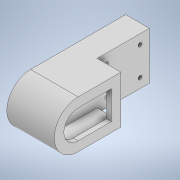
# Autodesk Inventor part: Link2_v2a
Saved by Autodesk Inventor 2022 (Build 260153000, 153)
## iProperties
Created: 2022-06-07
Part Number: Link2_v2a
Material: Generic
Document SubType Name: Modeling
Designer: Asus
Density: 1 g/cm^3
Appearance: Default
Author: Asus
Autodesk Inventor part; units mm, degrees
ref_plane "YZ Plane" through (0, 0, 0) normal (1, 0, 0) x (0, 1, 0)
ref_plane "XZ Plane" through (0, 0, 0) normal (0, 1, 0) x (-1, 0, 0)
ref_plane "XY Plane" through (0, 0, 0) normal (0, 0, 1) x (1, 0, 0)
sketch "Sketch1" plane through (0, 0, 0) normal (1, 0, 0) x (0, 1, 0)
  line L0 (25, 22.5) -> (-25, 22.5)
  line L1 (-25, 22.5) -> (-25, -100)
  line L2 (-25, -100) -> (25, -100)
  line L3 (25, -100) -> (25, 22.5)
  circle A0 centre (0, 0) radius 25
  circle A1 centre (0, 0) radius 20
  circle A2 centre (0, 0) radius 3.2936
  point P0 (25, 0)
  point P1 (-25, 0)
  dimension "d0" = 50
  dimension "d1" = 122.5
  dimension "d2" = 25
  dimension "d3" = 22.5
  dimension "d12" = 40
  dimension "d13" = 6.5872
  constraints: 8 end point, 3 centre point, 3 coincident, 2 parallel, 1 horizontal, 1 perpendicular, 1 tangent
  measures "d0" distance of L1.end L2.end
  measures "d1" distance of L0.end L1.end
  measures "d2" distance from line of L3 point (0, 0)
  measures "d3" distance from line of L0 point (0, 0)
  measures "d12" diameter of A1
  measures "d13" diameter of A2
extrude "Extrusion1" add sketch "Sketch1" along normal blind 5 contours A0 L0 | L0 A0 | L3 L2 L1 A0 | A1
sketch "Sketch4" plane through (5, 0, 0) normal (1, 0, 0) x (0, 0, -1)
  line L0 (100, -25) -> (100, 25) projected
  line L1 (100, 25) -> (0, 25) projected
  line L2 (100, -25) -> (0, -25)
  line L3 (0, -25) -> (0, 25)
  line L4 (0, 25) -> (100, 25)
  line L5 (100, 25) -> (100, -25)
  circle A0 centre (0, 0) radius 3.2936 projected
  arc A1 (15, 20) -> (15, -20) centre (0, 0) ccw
  circle A2 centre (0, 0) radius 20
  line L6 (0, 20) -> (95, 20)
  line L7 (95, 20) -> (95, -20)
  line L8 (95, -20) -> (0, -20)
  line L9 (0, -20) -> (0, 20)
  point P0 (0, -20)
  dimension "d15" = 40
  dimension "d14" = 50
  dimension "d16" = 5
  dimension "d17" = 5
  constraints: 16 end point, 4 parallel, 3 point on line, 2 coincident, 2 horizontal, 2 perpendicular, 2 point on circle, 1 centre point, 3 other
  measures "d14" diameter of A1
  measures "d16" distance between parallel lines of L2 L8
  measures "d17" distance between parallel lines of L0 L7
extrude "Extrusion3" add sketch "Sketch4" along normal blind 45 contours L2 A1 L8 L7 L6 L1 L0 | A1 L3 A2 | L3 L8 A1 | A1 L6 L3
sketch "Sketch5" plane through (50, 0, 0) normal (1, 0, 0) x (0, 0, -1)
  line L0 (100, -25) -> (100, 25) projected
  line L1 (0, 25) -> (100, 25)
  line L2 (100, 25) -> (100, -25)
  line L3 (100, -25) -> (0, -25)
  line L4 (0, -25) -> (0, 25)
  circle A0 centre (0, 0) radius 25
  arc A1 (0, 20) -> (0, -20) centre (0, 0) ccw projected
  circle A2 centre (0, 0) radius 15
  line L5 (0, 15) -> (35, 15)
  line L6 (35, 15) -> (35, -15)
  line L7 (35, -15) -> (0, -15)
  line L8 (0, -15) -> (0, 15)
  point P0 (0, -15)
  point P1 (100, 25)
  dimension "d20" = 30
  dimension "d21" = 10
  dimension "d22" = 50
  dimension "d23" = 35
  constraints: 16 end point, 4 parallel, 2 coincident, 2 horizontal, 2 perpendicular, 1 centre point, 1 point on line, 3 other
  measures "d21" distance between parallel lines of L3 L7
  measures "d22" diameter of A0
  measures "d23" distance from line of point (0, 0) L6
extrude "Extrusion4" add sketch "Sketch5" against normal blind 5 contours L3 A0 L7 L6 L5 L1 L0 | A0 L4 A1 | L4 L7 A0 | A0 L5 L4 | A1 L4 A2
sketch "Sketch6" plane through (5, 0, 0) normal (1, 0, 0) x (0, 0, -1)
  circle A0 centre (0, 0) radius 20
  line L0 (95, 20) -> (0, 20) projected
  line L1 (0, -20) -> (95, -20) projected
  line L2 (0, 20) -> (22, 20)
  line L3 (22, 20) -> (22, -20)
  line L4 (22, -20) -> (0, -20)
  line L5 (0, -20) -> (0, 20)
  dimension "d26" = 22
  constraints: 8 end point, 2 parallel, 1 centre point, 1 coincident, 1 horizontal, 1 perpendicular, 1 point on line
  measures "d26" distance between parallel lines of L3 L5
extrude "Extrusion5" add sketch "Sketch6" along normal blind 20
sketch "Sketch7" plane through (0, 0, 0) normal (-1, 0, 0) x (0, 0, 1)
  circle A0 centre (0, 0) radius 9.5
  dimension "d29" = 19
  constraints: 1 centre point, 1 coincident
  measures "d29" diameter of A0
extrude "Extrusion6" cut sketch "Sketch7" against normal blind 12.5
sketch "Sketch8" plane through (0, 0, 0) normal (-1, 0, 0) x (0, 0, 1)
  circle A0 centre (0, 0) radius 11.5
  dimension "d32" = 23
  constraints: 1 centre point, 1 coincident
  measures "d32" diameter of A0
extrude "Extrusion7" cut sketch "Sketch8" against normal blind 6.5
sketch "Sketch9" plane through (12.5, 0, 0) normal (-1, 0, 0) x (0, 0, 1)
  circle A0 centre (0, 0) radius 9.5 projected
  circle A1 centre (0, 0) radius 6.2
  line L0 (0, 0) -> (7.2952, 0)
  line L1 (0, 0) -> (-3.8354, 6.643)
  line L2 (0, 0) -> (-3.5239, -6.1036)
  circle A2 centre (-3.1, 5.3694) radius 1.45
  circle A3 centre (6.2, 0) radius 1.45
  circle A4 centre (-3.1, -5.3694) radius 1.45
  dimension "d35" = 12.4
  dimension "d36" = 120
  dimension "d37" = 120
  dimension "d38" = 2.9
  dimension "d39" = 2.9
  dimension "d40" = 2.9
  constraints: 6 end point, 4 centre point, 3 point on circle, 3 point on line, 1 coincident, 1 horizontal
  measures "d35" diameter of A1
  measures "d36" angle of L1 L0
  measures "d37" angle of L1 L2
  measures "d38" diameter of A2
  measures "d39" diameter of A3
  measures "d40" diameter of A4
extrude "Extrusion8" cut sketch "Sketch9" against normal blind 16 contours L0 A3 A1 | A1 A3 | A1 A3 L0 | A2 L1 A1 | A1 L1 A2 | A4 A1 | A1 L2 A4 | L1 A2 A1 | A1 A2 L1 | A1 A4 L2
sketch "Sketch10" plane through (25, 0, 0) normal (1, 0, 0) x (0, 0, -1)
  circle A0 centre (3.1, 5.3694) radius 1.45 projected
  circle A1 centre (3.1, 5.3694) radius 4
  circle A2 centre (3.1, -5.3694) radius 1.45 projected
  circle A3 centre (3.1, -5.3694) radius 4
  circle A4 centre (-6.2, 0) radius 1.45 projected
  circle A5 centre (-6.2, 0) radius 4
  point P0 (0, 0)
  dimension "d43" = 8
  dimension "d44" = 8
  dimension "d45" = 8
  constraints: 3 centre point, 3 coincident
  measures "d43" diameter of A5
  measures "d44" diameter of A3
  measures "d45" diameter of A1
extrude "Extrusion9" cut sketch "Sketch10" against normal blind 7
sketch "Sketch11" plane through (0, 25, 0) normal (0, 1, 0) x (1, 0, 0)
  line L0 (0, 100) -> (50, 100) projected
  line L1 (0, 100) -> (0, 0) projected
  line L2 (50, 100) -> (0, 100)
  line L3 (0, 100) -> (0, 45)
  line L4 (0, 45) -> (50, 45)
  line L5 (50, 45) -> (50, 100)
  line L6 (50, 0) -> (50, 100) projected
  line L7 (50, 100) -> (25, 100)
  line L8 (25, 100) -> (25, 45)
  line L9 (25, 45) -> (50, 45)
  line L10 (50, 45) -> (50, 100)
  dimension "d48" = 55
  constraints: 16 end point, 4 parallel, 2 horizontal, 2 perpendicular, 1 midpoint, 1 point on line
  measures "d48" distance between parallel lines of L0 L4
extrude "Extrusion10" cut sketch "Sketch11" against normal blind 50 contours L0 L5 L4 L8
sketch "Sketch12" plane through (5, 0, 0) normal (1, 0, 0) x (0, 0, -1)
  line L0 (95, 20) -> (22, 20) projected
  line L1 (22, -20) -> (95, -20) projected
  line L2 (95, 20) -> (45, 20)
  line L3 (45, 20) -> (45, -20)
  line L4 (45, -20) -> (95, -20)
  line L5 (95, -20) -> (95, 20)
  point P0 (0, 0)
  dimension "d51" = 50
  constraints: 8 end point, 2 parallel, 1 horizontal, 1 perpendicular, 1 point on line
  measures "d51" distance between parallel lines of L3 L5
extrude "Extrusion11" add sketch "Sketch12" along normal blind 20
sketch "Sketch13" plane through (25, 25, -45) normal (1, 0, 0) x (0, 0, -1)
  line L0 (10, -10) -> (45, -10)
  line L1 (45, -10) -> (45, -40)
  line L2 (45, -40) -> (10, -40)
  line L3 (10, -40) -> (10, -10)
  line L4 (0, 0) -> (55, 0) projected
  line L5 (55, 0) -> (55, -50) projected
  line L6 (55, -50) -> (0, -50) projected
  line L7 (0, -50) -> (0, 0) projected
  circle A0 centre (10, -10) radius 1.95
  circle A1 centre (10, -40) radius 1.95
  circle A2 centre (45, -40) radius 1.95
  circle A3 centre (45, -10) radius 1.95
  point P0 (-45, -25)
  dimension "d54" = 10
  dimension "d55" = 10
  dimension "d56" = 10
  dimension "d57" = 10
  dimension "d58" = 3.9
  dimension "d59" = 3.9
  dimension "d60" = 3.9
  dimension "d61" = 3.9
  constraints: 8 end point, 4 centre point, 4 coincident, 2 parallel, 1 horizontal, 1 perpendicular
  measures "d54" distance between parallel lines of L4 L0
  measures "d55" distance between parallel lines of L5 L1
  measures "d56" distance between parallel lines of L6 L2
  measures "d57" distance between parallel lines of L7 L3
  measures "d58" diameter of A0
  measures "d59" diameter of A3
  measures "d60" diameter of A2
  measures "d61" diameter of A1
extrude "Extrusion12" cut sketch "Sketch13" against normal blind 26 contours L3 A0 L0 | L0 A0 L3 | A3 L1 L0 | L0 L1 A3 | A1 L2 L3 | L3 L2 A1 | A2 L2 L1 | L1 L2 A2
sketch "Sketch14" plane through (0, 0, 0) normal (-1, 0, 0) x (0, 0, 1)
  circle A0 centre (-90, 15) radius 1.95 projected
  circle A1 centre (-90, 15) radius 4
  circle A2 centre (-55, 15) radius 1.95 projected
  circle A3 centre (-55, 15) radius 4
  circle A4 centre (-55, -15) radius 1.95 projected
  circle A5 centre (-55, -15) radius 4
  circle A6 centre (-90, -15) radius 1.95 projected
  circle A7 centre (-90, -15) radius 4
  point P0 (0, 0)
  dimension "d64" = 8
  dimension "d65" = 8
  dimension "d66" = 8
  dimension "d67" = 8
  constraints: 4 centre point, 4 coincident
  measures "d64" diameter of A1
  measures "d65" diameter of A3
  measures "d66" diameter of A5
  measures "d67" diameter of A7
extrude "Extrusion13" cut sketch "Sketch14" against normal blind 10 contours A0 | A1 | A2 | A3 | A5 | A7
sketch "Sketch15" plane through (5, 0, 0) normal (1, 0, 0) x (0, 0, -1)
  line L0 (45, -20) -> (45, 20) projected
  line L1 (22, -20) -> (45, -20) projected
  line L2 (45, 20) -> (22, 20)
  line L3 (22, 20) -> (22, -20)
  line L4 (22, -20) -> (45, -20)
  line L5 (45, -20) -> (45, 20)
  point P0 (0, 0)
  constraints: 8 end point, 2 parallel, 1 horizontal, 1 perpendicular
extrude "Extrusion14" add sketch "Sketch15" along normal blind 20
body "Solid1"
